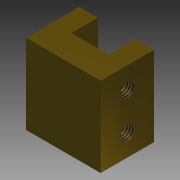
# Autodesk Inventor part: 13_0204_052
Saved by Autodesk Inventor 2012 SP1 (Build 160190100, 190)
## iProperties
Created: 2013-04-11
Part Number: 13_0204_052
Material: Default
Document SubType Name: Modeling
Designer: vogel
Density: 1 g/cm^3
Author: vogel
Autodesk Inventor part; units mm, degrees
ref_plane "YZ Plane" through (0, 0, 0) normal (1, 0, 0) x (0, 1, 0)
ref_plane "XZ Plane" through (0, 0, 0) normal (0, 1, 0) x (-1, 0, 0)
ref_plane "XY Plane" through (0, 0, 0) normal (0, 0, 1) x (1, 0, 0)
sketch "Skizze1" plane through (0, 0, 0) normal (0, 0, 1) x (1, 0, 0)
  line L0 (-9.8, 0) -> (9.8, 0) projected
  line L1 (0, -2) -> (0, 12) projected
  line L2 (-7, 0) -> (7, 0)
  line L3 (7, 0) -> (7, 10)
  line L4 (-7, 10) -> (-7, 0)
  line L5 (3.5, 10) -> (3.5, 5)
  line L6 (3.5, 5) -> (-3.5, 5)
  line L7 (-3.5, 5) -> (-3.5, 10)
  line L8 (7, 10) -> (3.5, 10)
  line L9 (-3.5, 10) -> (-7, 10)
  point P0 (0, 0)
  dimension "d0" = 10
  dimension "d1" = 5
  dimension "d3" = 3.5
  dimension "d6" = 7
  constraints: 16 end point, 4 parallel, 1 collinear, 1 horizontal, 1 perpendicular, 1 point on line, 2 other
  measures "d0" distance of L4.start L2.start
  measures "d1" distance between parallel lines of L0 L6
  measures "d3" distance of L7.end L4.start
  measures "d6" distance of L5.end L6.end
extrude "Extrusion1" add sketch "Skizze1" along normal blind 15
sketch "Skizze2" plane through (7, 0, 0) normal (1, 0, 0) x (0, 0, -1)
  line L0 (-15, 10) -> (-15, 0) projected
  line L1 (0, 0) -> (-15, 0) projected
  line L2 (0, 0) -> (0, 10) projected
  line L3 (-15, 5) -> (0, 5)
  point P0 (-11, 5)
  point P1 (-4, 5)
  dimension "d9" = 4
  dimension "d10" = 4
  dimension "d11" = 5
  constraints: 2 end point, 2 midpoint, 2 point on line, 1 perpendicular
  measures "d9" distance from line of L0 point (-11, 5)
  measures "d10" distance from line of L2 point (-4, 5)
  measures "d11" distance between parallel lines of L3 L1
hole "Bohrung1" at (7, 5, 11) at (7, 5, 4) direction (-1, 0, 0) diameter 2.459 end through all thread size "M3x0.5" class "6H" standard "ISO Metric profile"
